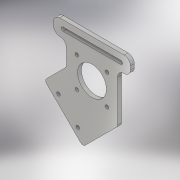
# Autodesk Inventor part: NEMA23MountPlatev2
Saved by Autodesk Inventor 2020.3 (Build 243373000, 373)
## iProperties
Created: 2021-09-06
Part Number: NEMA23MountPlatev2
Material: Aluminum 6061
Document SubType Name: Sheet Metal
Designer: justi
Density: 2.7 g/cm^3
Sheet Metal Rule: Default_mm
Appearance: Aluminum - Polished
Flat Pattern Width: 15.3848 cm
Flat Pattern Length: 13.2176 cm
Flat Pattern Area: 203.351 cm^2
Sheet Metal Width: 153.848 mm
Sheet Metal Length: 132.176 mm
Sheet Metal Area: 20335.134 mm^2
Author: justi
Autodesk Inventor part; units mm, degrees
ref_plane "YZ Plane" through (0, 0, 0) normal (1, 0, 0) x (0, 1, 0)
ref_plane "XZ Plane" through (0, 0, 0) normal (0, 1, 0) x (-1, 0, 0)
ref_plane "XY Plane" through (0, 0, 0) normal (0, 0, 1) x (1, 0, 0)
sketch "Sketch1" plane through (0, 0, 0) normal (0, 1, 0) x (-1, 0, 0)
  line L0 (40, 90) -> (-40, 90)
  line L1 (-40, 90) -> (-40, -81.7795)
  line L2 (40, -41.5685) -> (40, 90)
  line L3 (40, 90) -> (-40, -90) construction
  line L4 (-40, 90) -> (40, -90) construction
  circle A0 centre (-0.0013, 54.9992) radius 5.1
  line L5 (23.4987, -16.5008) -> (-23.5013, -16.5008) construction
  line L6 (-23.5013, -16.5008) -> (-23.5013, -63.5008) construction
  line L7 (-23.5013, -63.5008) -> (23.4987, -63.5008) construction
  line L8 (23.4987, -63.5008) -> (23.4987, -16.5008) construction
  line L9 (23.4987, -16.5008) -> (-23.5013, -63.5008) construction
  line L10 (-23.5013, -16.5008) -> (23.4987, -63.5008) construction
  circle A1 centre (23.4987, -16.5008) radius 2.75
  circle A2 centre (23.4987, -63.5008) radius 2.75
  circle A3 centre (-23.5013, -16.5008) radius 2.75
  circle A4 centre (-23.5013, -63.5008) radius 2.75
  line L11 (-0.0013, -90.0008) -> (-0.0013, -80) construction
  line L12 (19.9987, -11.0008) -> (-20.0013, -11.0008) construction
  line L13 (-20.0013, -11.0008) -> (-20.0013, -69.0008) construction
  line L14 (-20.0013, -69.0008) -> (19.9987, -69.0008) construction
  line L15 (19.9987, -69.0008) -> (19.9987, -11.0008) construction
  line L16 (19.9987, -11.0008) -> (-20.0013, -69.0008) construction
  line L17 (-20.0013, -11.0008) -> (19.9987, -69.0008) construction
  line L18 (-29.0013, -60.0008) -> (28.9987, -60.0008) construction
  line L19 (28.9987, -60.0008) -> (28.9987, -20.0008) construction
  line L20 (28.9987, -20.0008) -> (-29.0013, -20.0008) construction
  line L21 (-29.0013, -20.0008) -> (-29.0013, -60.0008)
  line L22 (-29.0013, -60.0008) -> (28.9987, -20.0008) construction
  line L23 (28.9987, -60.0008) -> (-29.0013, -20.0008) construction
  line L24 (-0.0013, 54.9992) -> (102.5291, -47.5313) construction
  line L25 (-0.0013, 54.9992) -> (144.9987, 54.9992) construction
  line L26 (28.2843, 83.2843) -> (-28.2843, 26.7157) construction
  line L27 (-28.2843, 26.7157) -> (74.2462, -75.8148) construction
  line L28 (74.2462, -75.8148) -> (130.8148, -19.2462) construction
  line L29 (130.8148, -19.2462) -> (28.2843, 83.2843) construction
  line L30 (28.2843, 83.2843) -> (74.2462, -75.8148) construction
  line L31 (-28.2843, 26.7157) -> (130.8148, -19.2462) construction
  line L32 (74.2462, -75.8148) -> (14.1407, -135.9202)
  line L33 (14.1407, -135.9202) -> (-0.0014, -121.7781)
  line L34 (-0.0014, -121.7781) -> (-31.7795, -90)
  line L35 (74.2462, -75.8148) -> (40, -41.5685)
  line L36 (-31.7795, -90) -> (-40, -81.7795)
  line L37 (44.1935, -105.8675) -> (37.1224, -98.7964)
  line L38 (37.1224, -98.7964) -> (52.1488, -83.7701) construction
  line L39 (37.1224, -98.7964) -> (22.096, -113.8228) construction
  circle A5 centre (52.1488, -83.7701) radius 2.75
  circle A6 centre (22.096, -113.8228) radius 2.75
  line L40 (-0.0013, 54.9992) -> (-0.0013, -40.0008)
  circle A7 centre (-0.0013, -40.0008) radius 22.5
  point P0 (0, 0)
  point P1 (51.2639, 3.7339)
  dimension "d0" = 80
  dimension "d1" = 180
  dimension "d3" = 10.2
  dimension "d5" = 47
  dimension "d6" = 47
  dimension "d7" = 5.5
  dimension "d8" = 5.5
  dimension "d9" = 5.5
  dimension "d10" = 5.5
  dimension "d12" = 40
  dimension "d13" = 58
  dimension "d14" = 58
  dimension "d15" = 40
  dimension "d27" = 45
  dimension "d28" = 145
  dimension "d29" = 80
  dimension "d30" = 145
  dimension "d31" = 85.002
  dimension "d32" = 20
  dimension "d33" = 10
  dimension "d35" = 21.2505
  dimension "d36" = 21.2505
  dimension "d37" = 5.5
  dimension "d38" = 5.5
  dimension "d53" = 95
  dimension "d54" = 45
  constraints: 82 end point, 10 parallel, 8 centre point, 7 coincident, 6 perpendicular, 5 horizontal, 5 midpoint, 3 point on line, 1 equal length, 1 vertical
  measures "d0" distance of L4.end L3.end
  measures "d1" distance of L3.end L0.end
  measures "d3" diameter of A0
  measures "d5" distance of L7.end L6.end
  measures "d6" distance of L6.end L5.end
  measures "d7" diameter of A1
  measures "d8" diameter of A2
  measures "d9" diameter of A3
  measures "d10" diameter of A4
  measures "d12" distance of L14.end L13.end
  measures "d13" distance of L13.end L12.end
  measures "d14" distance of L20.end L19.end
  measures "d15" distance of L19.end L18.end
  measures "d27" angle of L24 L25
  measures "d28" distance of L24.start L24.end
  measures "d29" distance of L28.end L27.end
  measures "d30" distance of L27.end L26.end
  measures "d31" distance of L27.end L32.end
  measures "d32" distance of L32.end L33.end
  measures "d33" distance of L37.start L37.end
  measures "d35" distance of L37.end L38.end
  measures "d36" distance of L37.end L39.end
  measures "d37" diameter of A5
  measures "d38" diameter of A6
  measures "d53" distance of L25.start L40.end
  measures "d54" diameter of A7
extrude "Plate3" add sketch "Sketch1" along normal blind 6
fillet "Fillet6" radius 5 4 edges at (-40, 3, -41.5685) (-74.2462, 3, -75.8148) (-14.1407, 3, -135.9202) (40, 3, -81.7795)
fillet "Fillet7" radius 40 2 edges at (40, 3, 90) (-40, 3, 90)
sketch "Sketch2" plane through (0, 0, 0) normal (0, -1, 0) x (1, 0, 0)
  circle A0 centre (0.0013, 54.9992) radius 5.1 projected
  line L0 (0.0013, 54.9992) -> (0.0013, -40.0008) construction
  line L1 (0.0013, 7.4992) -> (55.0013, 7.4992) construction
  line L2 (0.0013, 7.4992) -> (-54.9987, 7.4992) construction
  line L3 (-29.9987, 7.4992) -> (30.0013, 7.4992) construction
  line L4 (-29.9987, 4.7492) -> (30.0013, 4.7492)
  line L5 (30.0013, 10.2492) -> (-29.9987, 10.2492)
  arc A1 (-29.9987, 10.2492) -> (-29.9987, 4.7492) centre (-29.9987, 7.4992) ccw
  arc A2 (30.0013, 4.7492) -> (30.0013, 10.2492) centre (30.0013, 7.4992) ccw
  point P0 (0, 0)
  dimension "d43" = 95
  dimension "d44" = 55
  dimension "d45" = 55
  dimension "d46" = 30
  dimension "d47" = 5.5
  constraints: 14 end point, 4 point on circle, 4 tangent, 2 centre point, 2 horizontal, 2 midpoint, 1 parallel, 1 point on line, 1 vertical
  measures "d43" distance of L0.start L0.end
  measures "d44" distance of L1.start L1.end
  measures "d45" distance of L1.start L2.end
  measures "d46" distance of L1.start L3.end
  measures "d47" diameter of A2
extrude "Extrusion1" cut sketch "Sketch2" against normal blind 10 contours A1 L5 A2 L4
ref_plane "Work Plane2" through (30.0013, 0, 7.4992) normal (0, 0, -1) x (-1, 0, 0)
sketch "Sketch3" plane through (0, 0, 0) normal (0, -1, 0) x (1, 0, 0)
  line L0 (-29.9987, 4.7492) -> (30.0013, 4.7492) construction
  line L1 (0.0013, 4.7492) -> (0.0013, 10.2492) construction
  line L2 (30.0013, 10.2492) -> (-29.9987, 10.2492) construction
  point P0 (0, 0)
  constraints: 2 end point, 2 midpoint
sketch "Sketch4" plane through (0, 0, 0) normal (0, -1, 0) x (1, 0, 0)
  line L0 (-29.9987, 4.7492) -> (30.0013, 4.7492)
  line L1 (0.0013, 4.7492) -> (0.0013, 10.2492)
  line L2 (30.0013, 10.2492) -> (-29.9987, 10.2492)
  line L3 (-59.9987, 19.9992) -> (60.0013, 19.9992)
  line L4 (60.0013, 19.9992) -> (60.0013, -5.0008)
  line L5 (60.0013, -5.0008) -> (-59.9987, -5.0008)
  line L6 (-59.9987, -5.0008) -> (-59.9987, 19.9992)
  line L7 (-59.9987, 19.9992) -> (60.0013, -5.0008) construction
  line L8 (60.0013, 19.9992) -> (-59.9987, -5.0008) construction
  line L9 (-29.9987, 7.4992) -> (30.0013, 7.4992) construction
  line L10 (-29.9987, 4.7492) -> (30.0013, 4.7492)
  line L11 (30.0013, 10.2492) -> (-29.9987, 10.2492)
  arc A0 (-29.9987, 10.2492) -> (-29.9987, 4.7492) centre (-29.9987, 7.4992) ccw
  arc A1 (30.0013, 4.7492) -> (30.0013, 10.2492) centre (30.0013, 7.4992) ccw
  point P0 (0, 0)
  point P1 (0.0013, 7.4992)
  dimension "d56" = 120
  dimension "d57" = 25
  measures "d56" distance of L4.end L5.end
  measures "d57" distance of L3.end L4.end
sheet face with bend "Face4" sketch "Sketch4" thickness 6 toward (0, 1, 0) bend radius 6 relief straight relief width 6 relief depth 3
bend "Bend1"
fillet "Fillet11" radius 9.75 4 edges at (60.0013, 3, -5.0008) (60.0013, 3, 19.9992) (-59.9987, 3, -5.0008) (-59.9987, 3, 19.9992)
sketch "Sketch5" plane through (0, 0, 0) normal (0, -1, 0) x (1, 0, 0)
  line L0 (-29.9987, 4.7492) -> (30.0013, 4.7492) projected
  line L1 (0.0013, 4.7492) -> (0.0013, 10.2492)
  line L2 (30.0013, 10.2492) -> (-29.9987, 10.2492) projected
  line L3 (-44.9987, 7.4992) -> (45.0013, 7.4992) construction
  line L4 (-44.9987, 4.7492) -> (45.0013, 4.7492)
  line L5 (45.0013, 10.2492) -> (-44.9987, 10.2492)
  arc A0 (-44.9987, 10.2492) -> (-44.9987, 4.7492) centre (-44.9987, 7.4992) ccw
  arc A1 (45.0013, 4.7492) -> (45.0013, 10.2492) centre (45.0013, 7.4992) ccw
  point P0 (0, 0)
  point P1 (0.0013, 7.4992)
  dimension "d64" = 45
  dimension "d65" = 5.5
  constraints: 10 end point, 4 midpoint, 4 point on circle, 4 tangent, 2 centre point, 1 parallel, 1 perpendicular
  measures "d64" distance of point (0.001, 7.499) L3.end
  measures "d65" diameter of A1
extrude "Extrusion2" cut sketch "Sketch5" against normal blind 10
fillet "Fillet12" radius 9.75 4 edges at (40, 3, -5.0008) (-40, 3, -5.0008) (-40, 3, 19.9992) (40, 3, 19.9992)
sketch "Sketch6" plane through (0, 0, 0) normal (0, -1, 0) x (1, 0, 0)
  arc A0 (40, 29.7492) -> (49.75, 19.9992) centre (49.75, 29.7492) ccw projected
  arc A1 (-49.75, 19.9992) -> (-40, 29.7492) centre (-49.75, 29.7492) ccw projected
  line L0 (49.75, 19.9992) -> (-49.75, 19.9992)
  arc A2 (60.0013, 10.2492) -> (50.2513, 19.9992) centre (50.2513, 10.2492) ccw projected
  line L1 (50.2513, 19.9992) -> (-50.2487, 19.9992)
  line L2 (-50.2487, 19.9992) -> (-50.2487, 91.8023)
  line L3 (-50.2487, 91.8023) -> (50.2513, 91.8023)
  line L4 (50.2513, 91.8023) -> (50.2513, 19.9992)
  point P0 (0, 0)
  constraints: 10 end point, 2 horizontal, 2 parallel, 1 perpendicular, 1 tangent
extrude "Extrusion3" cut sketch "Sketch6" against normal through all
ref_plane "Work Plane3" through (-44.9987, 0, 7.4992) normal (0, 0, 1) x (1, 0, 0)
equation "\"d39\" = Thickness"
equation "\"BendRadius\" = Thickness"
equation "\"BendReliefWidth\" = Thickness"
equation "\"BendReliefDepth\" = 0.5 * Thickness"
equation "\"CornerReliefSize\" = 4 * Thickness"
equation "\"MinimumRemnant\" = 2 * Thickness"
equation "\"TransitionRadius\" = BendRadius"
equation "\"JacobiRadiusSize\" = BendRadius"
equation "\"GapSize\" = Thickness"
equation "\"Thickness\" = 6"
body "Solid3"
